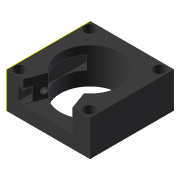
# Autodesk Inventor part: 00_NEMA23_holder
Saved by Autodesk Inventor 2019.4 (Build 234330000, 330)
## iProperties
Created: 2021-07-21
Part Number: 00_NEMA23_holder
Material: Generic
Document SubType Name: Modeling
Designer: diederichbenedict
Density: 1 g/cm^3
Appearance: Default
Author: diederichbenedict
Autodesk Inventor part; units mm, degrees
ref_plane "YZ Plane" through (0, 0, 0) normal (1, 0, 0) x (0, 1, 0)
ref_plane "XZ Plane" through (0, 0, 0) normal (0, 1, 0) x (-1, 0, 0)
ref_plane "XY Plane" through (0, 0, 0) normal (0, 0, 1) x (1, 0, 0)
sketch "Sketch1" plane through (0, 0, 0) normal (0, 1, 0) x (-1, 0, 0)
  line L0 (-28.2, -28.2) -> (28.2, -28.2)
  line L1 (28.2, -28.2) -> (28.2, 28.2)
  line L2 (28.2, 28.2) -> (-28.2, 28.2)
  line L3 (-28.2, 28.2) -> (-28.2, -28.2)
  line L4 (-28.2, -28.2) -> (28.2, 28.2) construction
  line L5 (28.2, -28.2) -> (-28.2, 28.2) construction
  line L6 (-23.55, 23.55) -> (23.55, 23.55) construction
  line L7 (23.55, 23.55) -> (23.55, -23.55) construction
  line L8 (23.55, -23.55) -> (-23.55, -23.55) construction
  line L9 (-23.55, -23.55) -> (-23.55, 23.55) construction
  line L10 (-23.55, 23.55) -> (23.55, -23.55) construction
  line L11 (23.55, 23.55) -> (-23.55, -23.55) construction
  circle A0 centre (23.55, 23.55) radius 2
  circle A1 centre (23.55, -23.55) radius 2
  circle A2 centre (-23.55, -23.55) radius 2
  circle A3 centre (-23.55, 23.55) radius 2
  circle A4 centre (0, 0) radius 20
  line L12 (28.2, 28.2) -> (-28.2, 28.2)
  line L13 (-28.2, 28.2) -> (-28.2, 38.2)
  line L14 (-28.2, 38.2) -> (28.2, 38.2)
  line L15 (28.2, 38.2) -> (28.2, 28.2)
  dimension "d0" = 56.4
  dimension "d1" = 56.4
  dimension "d2" = 47.1
  dimension "d3" = 47.1
  dimension "d4" = 4
  dimension "d5" = 4
  dimension "d6" = 4
  dimension "d7" = 4
  dimension "d8" = 40
  dimension "d16" = 10
  constraints: 32 end point, 6 parallel, 5 centre point, 5 coincident, 4 midpoint, 3 horizontal, 3 perpendicular
  measures "d0" distance of L2.end L1.end
  measures "d1" distance of L1.end L0.end
  measures "d2" distance of L7.end L8.end
  measures "d3" distance of L6.end L7.end
  measures "d4" diameter of A0
  measures "d5" diameter of A1
  measures "d6" diameter of A2
  measures "d7" diameter of A3
  measures "d8" diameter of A4
  measures "d16" distance of L12.end L13.end
extrude "Extrusion1" add sketch "Sketch1" along normal blind 24 contours L3 L2 L1 L0
sketch "Sketch2" plane through (0, 24, 0) normal (0, 1, 0) x (1, 0, 0)
  circle A0 centre (0, 0) radius 20 projected
  circle A1 centre (23.55, -23.55) radius 2 projected
  circle A2 centre (23.55, 23.55) radius 2 projected
  circle A3 centre (-23.55, 23.55) radius 2 projected
  circle A4 centre (-23.55, -23.55) radius 2 projected
  line L0 (28.2, 28.2) -> (-28.2, 28.2) projected
  line L1 (-28.2, 28.2) -> (-28.2, -28.2) projected
  line L2 (28.2, -28.2) -> (28.2, 28.2) projected
  circle A5 centre (0, 0) radius 6.5
  line L3 (-6.4978, 0.1686) -> (-26.2939, -54.2207)
  line L4 (-6.4978, 0.1686) -> (51.3822, 0.1686) construction
  line L5 (6.4521, -0.788) -> (25.9, -54.2207)
  line L6 (6.4521, -0.788) -> (63.314, -0.788) construction
  line L7 (25.9, -54.2207) -> (-26.2939, -54.2207)
  line L8 (-28.2, -28.2) -> (28.2, -28.2) projected
  dimension "d11" = 110
  dimension "d12" = 70
  dimension "d13" = 13
  constraints: 10 end point, 3 horizontal, 2 equal length, 2 point on circle, 1 centre point, 1 coincident
  measures "d11" angle of L3 L4
  measures "d12" angle of L5 L6
  measures "d13" diameter of A5
extrude "Extrusion2" cut sketch "Sketch2" against normal blind 15 contours L3 A5 L5 A0 | A0 L5 L8 L3 | A5 | L8 L5 L7 L3 picked at (-8.2958, -12.9873)
sketch "Sketch3" plane through (-28.2, 0, -28.2) normal (-1, 0, 0) x (0, 0, 1)
  line L0 (0, 0) -> (56.4, 0) projected
  line L1 (0, 24) -> (56.4, 24) projected
  line L2 (0, 0) -> (0, 24) projected
  line L3 (49.75, 24) -> (53.75, 24) projected
  line L4 (53.75, 0) -> (49.75, 0) projected
  line L5 (2.65, 24) -> (6.65, 24) projected
  line L6 (6.65, 0) -> (2.65, 0) projected
  line L7 (6.65, 0) -> (6.65, 24) projected
  line L8 (2.65, 0) -> (2.65, 24) projected
  line L9 (49.75, 0) -> (49.75, 24) projected
  line L10 (53.75, 0) -> (53.75, 24) projected
  line L11 (56.4, 0) -> (56.4, 24) projected
  point P0 (28.2, 0)
sketch "Sketch4" plane through (-28.2, 0, -28.2) normal (-1, 0, 0) x (0, 0, 1)
  line L0 (0, 0) -> (56.4, 0) projected
  line L1 (0, 24) -> (56.4, 24) projected
  line L2 (0, 0) -> (0, 24) projected
  circle A0 centre (4, 14) radius 2.5
  circle A1 centre (46, 14) radius 2.5
  line L3 (4.5098, 0) -> (4.5098, 24) construction
  line L4 (0, 24) -> (66.4, 24) construction
  line L5 (56.4, 0) -> (56.4, 24) projected
  point P0 (28.2, 0)
  dimension "d17" = 5
  dimension "d18" = 5
  dimension "d19" = 4.5098
  dimension "d20" = 4
  dimension "d21" = 14
  dimension "d22" = 0
  dimension "d23" = 42
  constraints: 2 centre point, 2 end point, 2 point on line, 1 parallel
  measures "d17" diameter of A0
  measures "d18" diameter of A1
  measures "d19" distance between parallel lines of L3 L2
  measures "d20" distance from line of A0.centre L2
  measures "d21" distance from line of A0.centre L0
  measures "d22" vertical distance of A1.centre A0.centre
  measures "d23" distance of A1.centre A0.centre
hole "Hole1" at (-28.2, 14, -24.2) at (-28.2, 14, 17.8) direction (1, 0, 0) diameter 4 depth 16 tip angle 118
sketch "Sketch5" plane through (0, 24, 0) normal (0, 1, 0) x (1, 0, 0)
  line L0 (-16.8232, -28.2) -> (-12.2994, -15.771) projected
  arc A0 (11.9912, -16.0066) -> (-12.2994, -15.771) centre (0, 0) ccw projected
  line L1 (11.9912, -16.0066) -> (16.4292, -28.2) projected
  line L2 (28.2, -28.2) -> (28.2, 28.2) projected
  line L3 (28.2, 28.2) -> (-28.2, 28.2) projected
  line L4 (-28.2, 28.2) -> (-28.2, -28.2) projected
  circle A1 centre (23.55, -23.55) radius 2 projected
  circle A2 centre (23.55, 23.55) radius 2 projected
  circle A3 centre (-23.55, 23.55) radius 2 projected
  circle A4 centre (-23.55, -23.55) radius 2 projected
  line L5 (16.4292, -28.2) -> (28.2, -28.2) projected
  line L6 (-28.2, -28.2) -> (-16.8232, -28.2) projected
hole "Hole2" at (-23.55, 24, 23.55) at (-23.55, 24, -23.55) at (23.55, 24, -23.55) at (23.55, 24, 23.55) direction (0, -1, 0) diameter 4 depth 12 tip angle 118 counterbore diameter 8 counterbore depth 10
sketch "Sketch6" plane through (28.2, 0, -28.2) normal (0, 0, -1) x (-1, 0, 0)
  line L0 (41.2379, 16) -> (56.4, 16) projected
  line L1 (40.4, 12) -> (56.4, 12) projected
  line L2 (48.3294, 18.4358) -> (43.3294, 18.4358)
  line L3 (43.3294, 18.4358) -> (43.3294, 9.4358)
  line L4 (43.3294, 9.4358) -> (48.3294, 9.4358)
  line L5 (48.3294, 9.4358) -> (48.3294, 18.4358)
  line L6 (48.3294, 18.4358) -> (43.3294, 9.4358) construction
  line L7 (43.3294, 18.4358) -> (48.3294, 9.4358) construction
  point P0 (28.2, 0)
  point P1 (45.8294, 13.9358)
  dimension "d38" = 9
  dimension "d39" = 5
  constraints: 12 end point, 2 midpoint, 2 parallel, 1 horizontal, 1 perpendicular
  measures "d38" distance between parallel lines of L4 L2
  measures "d39" distance between parallel lines of L3 L5
extrude "Extrusion3" cut sketch "Sketch6" against normal through all
body "Solid1"
